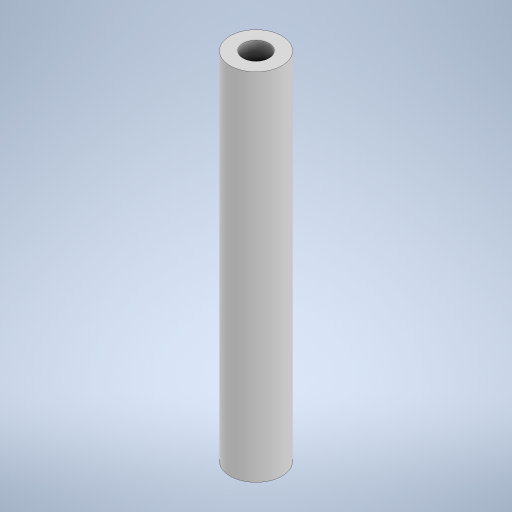
# Autodesk Inventor part: MountScrew_test
Saved by Autodesk Inventor 2024.2 (Build 282272000, 272)
## iProperties
Created: 2024-04-16
Part Number: MountScrew_test
Material: Generic
Document SubType Name: Modeling
Designer: ringl
Density: 1 g/cm^3
Appearance: Default
Author: ringl
Autodesk Inventor part; units mm, degrees
ref_plane "YZ Plane" through (0, 0, 0) normal (1, 0, 0) x (0, 1, 0)
ref_plane "XZ Plane" through (0, 0, 0) normal (0, 1, 0) x (-1, 0, 0)
ref_plane "XY Plane" through (0, 0, 0) normal (0, 0, 1) x (1, 0, 0)
sketch "Sketch1" plane through (0, 0, 0) normal (0, 1, 0) x (-1, 0, 0)
  circle A0 centre (0, 0) radius 4
  circle A1 centre (0, 0) radius 2.6
  dimension "d0" = 8
  dimension "d1" = 5.2
  constraints: 2 centre point, 2 coincident
  measures "d0" diameter of A0
  measures "d1" diameter of A1
extrude "Extrusion1" add sketch "Sketch1" along normal blind 5
sketch "Sketch2" plane through (0, 5, 0) normal (0, 1, 0) x (1, 0, 0)
  circle A0 centre (0, 0) radius 4 projected
  circle A1 centre (0, 0) radius 1.5
  circle A2 centre (0, 0) radius 4
  dimension "d4" = 3
  dimension "d5" = 8
  constraints: 2 centre point, 2 coincident
  measures "d4" diameter of A1
  measures "d5" diameter of A2
extrude "Extrusion2" add sketch "Sketch2" along normal blind 50
sketch "Sketch3" plane through (0, 55, 0) normal (0, 1, 0) x (1, 0, 0)
  circle A0 centre (0, 0) radius 2
  dimension "d8" = 4
  constraints: 1 centre point, 1 coincident
  measures "d8" diameter of A0
extrude "Extrusion3" cut sketch "Sketch3" against normal blind 5
body "Solid1"
